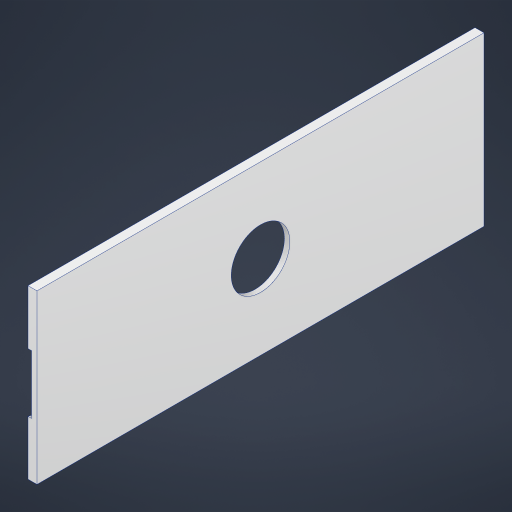
# Autodesk Inventor part: Osnova
Saved by Autodesk Inventor 2024 (Build 280153000, 153)
## iProperties
Created: 2023-12-23
Part Number: Osnova
Material: Aluminum 6061
Document SubType Name: Modeling
Designer: KirikDK
Mass: 1764.86 g
Surface Area: 1962.99 cm^2
Volume: 653.653 cm^3
Density: 2.7 g/cm^3
Appearance: Aluminum - Flat
Author: KirikDK
Autodesk Inventor part; units mm, degrees
ref_plane "YZ Plane" through (0, 0, 0) normal (1, 0, 0) x (0, 1, 0)
ref_plane "XZ Plane" through (0, 0, 0) normal (0, 1, 0) x (-1, 0, 0)
ref_plane "XY Plane" through (0, 0, 0) normal (0, 0, 1) x (1, 0, 0)
sketch "Sketch1" plane through (0, 0, 0) normal (0, 1, 0) x (-1, 0, 0)
  line L0 (95, 271.4286) -> (85, 271.4286)
  line L1 (85, 271.4286) -> (85, -224.5714)
  line L2 (85, -224.5714) -> (95, -224.5714)
  line L3 (95, -224.5714) -> (95, 271.4286)
  point P0 (0, 0)
  dimension "d0" = 10
  dimension "d1" = 496
  constraints: 8 end point, 2 parallel, 1 horizontal, 1 perpendicular
  measures "d0" distance of L0.start L0.end
  measures "d1" distance of L2.end L0.start
extrude "Extrusion1" add sketch "Sketch1" along normal blind 186
sketch "Sketch3" plane through (-85, 0, 271.4286) normal (1, 0, 0) x (0, 0, -1)
  line L0 (0, 0) -> (496, 0) projected
  line L1 (496, 0) -> (496, 186) projected
  line L2 (0, 186) -> (496, 186) projected
  line L3 (0, 0) -> (0, 186) projected
  circle A0 centre (0, 93) radius 5
  line L4 (0, 0) -> (496, 0) projected
  circle A1 centre (248, 0) radius 5
  line L5 (0, 0) -> (248, 0)
  line L6 (0, 93) -> (0, 0)
  circle A2 centre (248, 93) radius 32.5
  point P0 (271.4286, 0)
  dimension "d16" = 65
  dimension "d19" = 93
  dimension "d20" = 248
  dimension "d21" = 248
  dimension "d22" = 93
  constraints: 4 end point, 3 centre point, 3 midpoint, 1 horizontal
  measures "d16" diameter of A2
  measures "d19" distance of point (248, 0) A2.centre
  measures "d20" distance from line of L3 A2.centre
  measures "d21" distance from line of L1 A2.centre
  measures "d22" distance from line of L2 A2.centre
extrude "Extrusion5" cut sketch "Sketch3" against normal blind 186 contours A2
sketch "Sketch5" plane through (-95, 0, -224.5714) normal (-1, 0, 0) x (0, 0, 1)
  circle A0 centre (248, 93) radius 32.5 projected
  circle A1 centre (248, 93) radius 90.5
  line L0 (0, 0) -> (0, 186) projected
  circle A2 centre (0, 93) radius 32.5
  line L1 (496, 0) -> (496, 186) projected
  circle A3 centre (496, 93) radius 32.5
  line L2 (0, 60.5) -> (226.495, 5.0922)
  line L3 (0, 125.5) -> (224.5714, 180.4148)
  line L4 (496, 125.5) -> (269.505, 180.9078)
  line L5 (496, 60.5) -> (271.4286, 5.5852)
  point P0 (224.5714, 0)
  dimension "d23" = 181
  constraints: 8 end point, 8 point on circle, 4 point on line, 3 centre point, 2 midpoint, 2 parallel, 1 coincident, 1 tangent
  measures "d23" diameter of A1
extrude "Extrusion6" cut sketch "Sketch5" against normal blind 4 contours A1 | A1 L4 A3 L5 | A1 L2 A2 L3 | L1 A3 | A2 L0 picked at (485.2457, 91.6942) picked at (6.7545, 84.5302)
body "Solid1"
